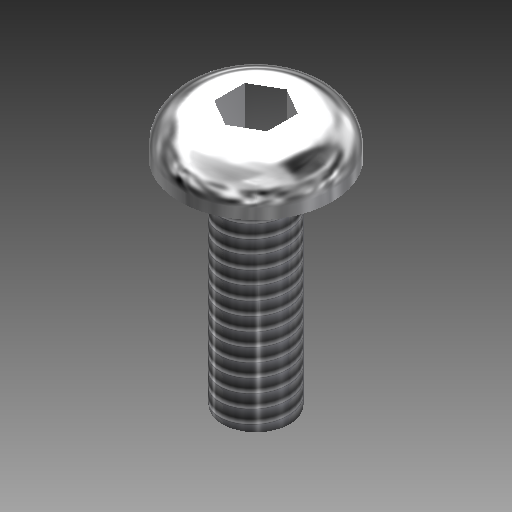
# Autodesk Inventor part: m3x8
Saved by Autodesk Inventor 2018 (Build 220112000, 112)
## iProperties
Created: 2013-08-30
Part Number: m3x8
Material: Generic
Document SubType Name: Modeling
Designer: Admin
Density: 1 g/cm^3
Appearance: Default
Author: Admin
Autodesk Inventor part; units mm, degrees
ref_plane "YZ Plane" through (0, 0, 0) normal (1, 0, 0) x (0, 1, 0)
ref_plane "XZ Plane" through (0, 0, 0) normal (0, 1, 0) x (-1, 0, 0)
ref_plane "XY Plane" through (0, 0, 0) normal (0, 0, 1) x (1, 0, 0)
sketch "Sketch1" plane through (0, 0, 0) normal (0, 1, 0) x (-1, 0, 0)
  circle A0 centre (0, 0) radius 1.2573
  dimension "d0" = 2.5146
  constraints: 1 centre point, 1 coincident
  measures "d0" diameter of A0
extrude "Extrusion1" add sketch "Sketch1" against normal blind 8
sketch "Sketch2" plane through (0, 0, 0) normal (0, 1, 0) x (1, 0, 0)
  circle A0 centre (0, 0) radius 1.2573 projected
  circle A1 centre (0, 0) radius 2.8448
  line L0 (0, 0) -> (0.9906, 0)
  line L1 (0.9906, -0.5719) -> (0, -1.1438)
  line L2 (0, -1.1438) -> (-0.9906, -0.5719)
  line L3 (-0.9906, -0.5719) -> (-0.9906, 0.5719)
  line L4 (-0.9906, 0.5719) -> (0, 1.1438)
  line L5 (0, 1.1438) -> (0.9906, 0.5719)
  line L6 (0.9906, 0.5719) -> (0.9906, -0.5719)
  dimension "d7" = 0.9906
  constraints: 14 end point, 2 coincident, 1 centre point, 1 horizontal, 1 midpoint, 13 other
  measures "d7" distance of L0.start L0.end
extrude "Extrusion2" add sketch "Sketch2" along normal blind 1.651 contours A0 | A1
fillet "Fillet1" radius 1.27 1 edges at (-2.8448, 1.651, 0)
thread "Thread1" size "M3x0.5" class "6g" standard "ANSI Metric M Profile" full length
body "Solid1"
